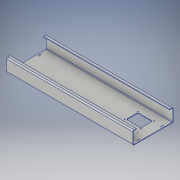
# Autodesk Inventor part: main chassis
Saved by Autodesk Inventor 2018.1 (Build 221171000, 171)
## iProperties
Created: 2018-11-08
Part Number: main chassis
Material: Aluminum 6061
Document SubType Name: Sheet Metal
Designer: RCCol
Density: 2.7 g/cm^3
Sheet Metal Rule: .125 thick aluminum
Appearance: Aluminum - Flat
Author: RCCol
Autodesk Inventor part; units mm, degrees
ref_plane "YZ Plane" through (0, 0, 0) normal (1, 0, 0) x (0, 1, 0)
ref_plane "XZ Plane" through (0, 0, 0) normal (0, 1, 0) x (-1, 0, 0)
ref_plane "XY Plane" through (0, 0, 0) normal (0, 0, 1) x (1, 0, 0)
sketch "Sketch1" plane through (0, 0, 0) normal (0, 1, 0) x (-1, 0, 0)
  line L0 (0, 0) -> (-673.1, 0)
  line L1 (-673.1, 0) -> (-673.1, -215.9)
  line L2 (-673.1, -215.9) -> (0, -215.9)
  line L3 (0, -215.9) -> (0, 0)
  dimension "d0" = 673.1
  dimension "d1" = 215.9
  measures "d0" distance of L2.end L1.end
  measures "d1" distance of L1.end L0.end
extrude "Plate1" add sketch "Sketch1" along normal blind 3.175
sketch "Sketch2" plane through (0, 0, -212.725) normal (0, 0, -1) x (-1, 0, 0)
  line L0 (-673.1, 0) -> (0, 0)
  line L1 (0, 0) -> (0, 69.85)
  line L2 (0, 69.85) -> (-673.1, 69.85)
  line L3 (-673.1, 69.85) -> (-673.1, 0)
  constraints: 6 end point, 1 horizontal, 1 perpendicular, 1 vertical
edge flange "Flange1" height 69.85 angle 90 thickness 3.175 bend radius 3.175 thickness toward (0, 0, -1) relief straight relief width 3.175 relief depth 1.5875 edges at (336.55, 3.175, -215.9) wall of the first edge with corners at (673.1, 0, -212.725) (0, 0, -212.725) (0, 69.85, -212.725) (673.1, 69.85, -212.725)
bend "Bend1"
corner "Corner1"
sketch "Sketch3" plane through (673.1, 0, -3.175) normal (0, 0, 1) x (1, 0, 0)
  line L0 (-673.1, 0) -> (0, 0)
  line L1 (0, 0) -> (0, 69.85)
  line L2 (0, 69.85) -> (-673.1, 69.85)
  line L3 (-673.1, 69.85) -> (-673.1, 0)
  constraints: 6 end point, 1 horizontal, 1 perpendicular, 1 vertical
edge flange "Flange2" height 69.85 angle 90 thickness 3.175 bend radius 3.175 thickness toward (0, 0, 1) relief straight relief width 3.175 relief depth 1.5875 edges at (336.55, 3.175, 0) wall of the first edge with corners at (0, 0, -3.175) (673.1, 0, -3.175) (673.1, 69.85, -3.175) (0, 69.85, -3.175)
bend "Bend2"
corner "Corner2"
sketch "Sketch4" plane through (0, 66.675, -215.9) normal (0, 1, 0) x (-1, 0, 0)
  line L0 (-673.1, 0) -> (0, 0)
  line L1 (0, 0) -> (0, 19.05)
  line L2 (0, 19.05) -> (-673.1, 19.05)
  line L3 (-673.1, 19.05) -> (-673.1, 0)
  constraints: 6 end point, 1 horizontal, 1 perpendicular, 1 vertical
edge flange "Flange3" height 19.05 angle 90 thickness 3.175 bend radius 3.175 thickness toward (0, 1, 0) relief straight relief width 3.175 relief depth 1.5875 corner gap 3.175 corner form 0 edges at (336.55, 69.85, -212.725) (336.55, 69.85, -3.175) wall of the first edge with corners at (673.1, 66.675, -215.9) (0, 66.675, -215.9) (0, 66.675, -196.85) (673.1, 66.675, -196.85)
bend "Bend3"
corner "Corner3"
sketch "A$C12E85A68" plane through (0, 0, 0) normal (0, 0, 1) x (1, 0, 0)
  line L0 (6.985, 0) -> (-6.985, 0)
  point P0 (0, 0)
sketch "A$C3FBB3793" plane through (0, 0, 0) normal (0, 0, 1) x (1, 0, 0)
  line L0 (6.985, 0) -> (-6.985, 0)
  point P0 (0, 0)
sketch "switch" plane through (0, 0, 0) normal (0, 0, 1) x (1, 0, 0)
  circle A0 centre (258.1551, -160.6447) radius 1.9558
  circle A1 centre (258.1551, -132.0697) radius 1.9558
  line L0 (261.3301, -152.7072) -> (254.9801, -152.7072)
  line L1 (254.9801, -152.7072) -> (254.9801, -140.0072)
  line L2 (254.9801, -140.0072) -> (261.3301, -140.0072)
  line L3 (261.3301, -140.0072) -> (261.3301, -152.7072)
  point P0 (0, 0)
sketch "A$C150B116C" plane through (0, 0, 0) normal (0, 0, 1) x (1, 0, 0)
  circle A0 centre (0, -14.2875) radius 1.9558
  circle A1 centre (0, 14.2875) radius 1.9558
  line L0 (3.175, -6.35) -> (-3.175, -6.35)
  line L1 (-3.175, -6.35) -> (-3.175, 6.35)
  line L2 (-3.175, 6.35) -> (3.175, 6.35)
  line L3 (3.175, 6.35) -> (3.175, -6.35)
  point P0 (0, 0)
sketch "A$C47CC5A6E" plane through (0, 0, 0) normal (0, 0, 1) x (1, 0, 0)
  circle A0 centre (0, -14.2875) radius 1.9558
  circle A1 centre (0, 14.2875) radius 1.9558
  line L0 (3.175, -6.35) -> (-3.175, -6.35)
  line L1 (-3.175, -6.35) -> (-3.175, 6.35)
  line L2 (-3.175, 6.35) -> (3.175, 6.35)
  line L3 (3.175, 6.35) -> (3.175, -6.35)
  point P0 (0, 0)
sketch "A$C2A516532" plane through (0, 0, 0) normal (0, 0, 1) x (1, 0, 0)
  circle A0 centre (0, -14.2875) radius 1.9558
  circle A1 centre (0, 14.2875) radius 1.9558
  line L0 (3.175, -6.35) -> (-3.175, -6.35)
  line L1 (-3.175, -6.35) -> (-3.175, 6.35)
  line L2 (-3.175, 6.35) -> (3.175, 6.35)
  line L3 (3.175, 6.35) -> (3.175, -6.35)
  point P0 (0, 0)
sketch "A$C2A9E7CC2" plane through (0, 0, 0) normal (0, 0, 1) x (1, 0, 0)
  circle A0 centre (0, -12.7) radius 4.7625
  circle A1 centre (0, 12.7) radius 4.7625
  circle A2 centre (0, 12.7) radius 4.7625
  circle A3 centre (0, -12.7) radius 4.7625
  point P0 (0, 0)
sketch "A$C56AF9537" plane through (0, 0, 0) normal (0, 0, 1) x (1, 0, 0)
  circle A0 centre (0, 0) radius 4.7625
  circle A1 centre (38.1, 0) radius 4.7625
  circle A2 centre (38.1, 0) radius 4.7625
  circle A3 centre (0, 0) radius 4.7625
sketch "A$C5AAF1D81" plane through (0, 0, 0) normal (0, 0, 1) x (1, 0, 0)
  circle A0 centre (0, 0) radius 4.7625
sketch "A$C295C71F8" plane through (0, 0, 0) normal (0, 0, 1) x (1, 0, 0)
  line L0 (-24.6482, -5.1614) -> (-26.1518, -5.1614)
  arc A0 (-24.6482, -6.1774) -> (-26.1518, -6.1774) centre (-25.4, 0) ccw
  line L1 (-26.1518, -5.1614) -> (-26.1518, -6.1774)
  line L2 (-24.6482, -6.1774) -> (-24.6482, -5.1614)
  line L3 (0.7518, -5.1614) -> (-0.7518, -5.1614)
  arc A1 (0.7518, -6.1774) -> (-0.7518, -6.1774) centre (0, 0) ccw
  line L4 (-0.7518, -5.1614) -> (-0.7518, -6.1774)
  line L5 (0.7518, -6.1774) -> (0.7518, -5.1614)
sketch "A$C1F257043" plane through (0, 0, 0) normal (0, 0, 1) x (1, 0, 0)
  line L0 (-24.6482, -5.1614) -> (-26.1518, -5.1614)
  arc A0 (-24.6482, -6.1774) -> (-26.1518, -6.1774) centre (-25.4, 0) ccw
  line L1 (-26.1518, -5.1614) -> (-26.1518, -6.1774)
  line L2 (-24.6482, -6.1774) -> (-24.6482, -5.1614)
  line L3 (0.7518, -5.1614) -> (-0.7518, -5.1614)
  arc A1 (0.7518, -6.1774) -> (-0.7518, -6.1774) centre (0, 0) ccw
  line L4 (-0.7518, -5.1614) -> (-0.7518, -6.1774)
  line L5 (0.7518, -6.1774) -> (0.7518, -5.1614)
sketch "A$C62022436" plane through (0, 0, 0) normal (0, 0, 1) x (1, 0, 0)
  circle A0 centre (0, 0) radius 3.2004
sketch "A$C5D572602" plane through (0, 0, 0) normal (0, 0, 1) x (1, 0, 0)
  circle A0 centre (237.6, 34.925) radius 15.1
  arc A1 (239.251, 56.7808) -> (238.6557, 57.3761) centre (238.6557, 56.7808) ccw
  arc A2 (238.6557, 52.4739) -> (239.251, 53.0692) centre (238.6557, 53.0692) ccw
  line L0 (239.251, 53.0692) -> (239.251, 56.7808)
  arc A3 (236.5443, 57.3761) -> (235.949, 56.7808) centre (236.5443, 56.7808) ccw
  line L1 (235.949, 53.0692) -> (235.949, 56.7808)
  line L2 (238.6557, 57.3761) -> (236.5443, 57.3761)
  line L3 (238.6557, 52.4739) -> (236.5443, 52.4739)
  arc A4 (235.949, 53.0692) -> (236.5443, 52.4739) centre (236.5443, 53.0692) ccw
  arc A5 (239.251, 16.7808) -> (238.6557, 17.3761) centre (238.6557, 16.7808) ccw
  arc A6 (238.6557, 12.4739) -> (239.251, 13.0692) centre (238.6557, 13.0692) ccw
  line L4 (239.251, 13.0692) -> (239.251, 16.7808)
  arc A7 (236.5443, 17.3761) -> (235.949, 16.7808) centre (236.5443, 16.7808) ccw
  line L5 (235.949, 13.0692) -> (235.949, 16.7808)
  line L6 (238.6557, 17.3761) -> (236.5443, 17.3761)
  line L7 (238.6557, 12.4739) -> (236.5443, 12.4739)
  arc A8 (235.949, 13.0692) -> (236.5443, 12.4739) centre (236.5443, 13.0692) ccw
  circle A9 centre (174.1, 34.925) radius 15.1
  arc A10 (175.751, 56.7808) -> (175.1557, 57.3761) centre (175.1557, 56.7808) ccw
  arc A11 (175.1557, 52.4739) -> (175.751, 53.0692) centre (175.1557, 53.0692) ccw
  line L8 (175.751, 53.0692) -> (175.751, 56.7808)
  arc A12 (173.0443, 57.3761) -> (172.449, 56.7808) centre (173.0443, 56.7808) ccw
  line L9 (172.449, 53.0692) -> (172.449, 56.7808)
  line L10 (175.1557, 57.3761) -> (173.0443, 57.3761)
  line L11 (175.1557, 52.4739) -> (173.0443, 52.4739)
  arc A13 (172.449, 53.0692) -> (173.0443, 52.4739) centre (173.0443, 53.0692) ccw
  arc A14 (175.751, 16.7808) -> (175.1557, 17.3761) centre (175.1557, 16.7808) ccw
  arc A15 (175.1557, 12.4739) -> (175.751, 13.0692) centre (175.1557, 13.0692) ccw
  line L12 (175.751, 13.0692) -> (175.751, 16.7808)
  arc A16 (173.0443, 17.3761) -> (172.449, 16.7808) centre (173.0443, 16.7808) ccw
  line L13 (172.449, 13.0692) -> (172.449, 16.7808)
  line L14 (175.1557, 17.3761) -> (173.0443, 17.3761)
  line L15 (175.1557, 12.4739) -> (173.0443, 12.4739)
  arc A17 (172.449, 13.0692) -> (173.0443, 12.4739) centre (173.0443, 13.0692) ccw
  circle A18 centre (110.6, 34.925) radius 15.1
  arc A19 (112.251, 56.7808) -> (111.6557, 57.3761) centre (111.6557, 56.7808) ccw
  arc A20 (111.6557, 52.4739) -> (112.251, 53.0692) centre (111.6557, 53.0692) ccw
  line L16 (112.251, 53.0692) -> (112.251, 56.7808)
  arc A21 (109.5443, 57.3761) -> (108.949, 56.7808) centre (109.5443, 56.7808) ccw
  line L17 (108.949, 53.0692) -> (108.949, 56.7808)
  line L18 (111.6557, 57.3761) -> (109.5443, 57.3761)
  line L19 (111.6557, 52.4739) -> (109.5443, 52.4739)
  arc A22 (108.949, 53.0692) -> (109.5443, 52.4739) centre (109.5443, 53.0692) ccw
  arc A23 (112.251, 16.7808) -> (111.6557, 17.3761) centre (111.6557, 16.7808) ccw
  arc A24 (111.6557, 12.4739) -> (112.251, 13.0692) centre (111.6557, 13.0692) ccw
  line L20 (112.251, 13.0692) -> (112.251, 16.7808)
  arc A25 (109.5443, 17.3761) -> (108.949, 16.7808) centre (109.5443, 16.7808) ccw
  line L21 (108.949, 13.0692) -> (108.949, 16.7808)
  line L22 (111.6557, 17.3761) -> (109.5443, 17.3761)
  line L23 (111.6557, 12.4739) -> (109.5443, 12.4739)
  arc A26 (108.949, 13.0692) -> (109.5443, 12.4739) centre (109.5443, 13.0692) ccw
  circle A27 centre (47.1, 34.925) radius 15.1
  arc A28 (48.751, 56.7808) -> (48.1557, 57.3761) centre (48.1557, 56.7808) ccw
  arc A29 (48.1557, 52.4739) -> (48.751, 53.0692) centre (48.1557, 53.0692) ccw
  line L24 (48.751, 53.0692) -> (48.751, 56.7808)
  arc A30 (46.0443, 57.3761) -> (45.449, 56.7808) centre (46.0443, 56.7808) ccw
  line L25 (45.449, 53.0692) -> (45.449, 56.7808)
  line L26 (48.1557, 57.3761) -> (46.0443, 57.3761)
  line L27 (48.1557, 52.4739) -> (46.0443, 52.4739)
  arc A31 (45.449, 53.0692) -> (46.0443, 52.4739) centre (46.0443, 53.0692) ccw
  arc A32 (48.751, 16.7808) -> (48.1557, 17.3761) centre (48.1557, 16.7808) ccw
  arc A33 (48.1557, 12.4739) -> (48.751, 13.0692) centre (48.1557, 13.0692) ccw
  line L28 (48.751, 13.0692) -> (48.751, 16.7808)
  arc A34 (46.0443, 17.3761) -> (45.449, 16.7808) centre (46.0443, 16.7808) ccw
  line L29 (45.449, 13.0692) -> (45.449, 16.7808)
  line L30 (48.1557, 17.3761) -> (46.0443, 17.3761)
  line L31 (48.1557, 12.4739) -> (46.0443, 12.4739)
  arc A35 (45.449, 13.0692) -> (46.0443, 12.4739) centre (46.0443, 13.0692) ccw
  circle A36 centre (269.35, 26.3058) radius 1.651
  circle A37 centre (450.85, 36.5125) radius 9.525
  circle A38 centre (440.7472, 46.6153) radius 1.651
  circle A39 centre (460.9528, 26.4097) radius 1.651
  circle A40 centre (412.75, 36.5125) radius 9.525
  circle A41 centre (402.6472, 46.6153) radius 1.651
  circle A42 centre (422.8528, 26.4097) radius 1.651
  circle A43 centre (374.65, 36.5125) radius 9.525
  circle A44 centre (364.5472, 46.6153) radius 1.651
  circle A45 centre (384.7528, 26.4097) radius 1.651
  circle A46 centre (336.55, 36.5125) radius 9.525
  circle A47 centre (326.4472, 46.6153) radius 1.651
  circle A48 centre (346.6528, 26.4097) radius 1.651
  circle A49 centre (298.45, 36.5125) radius 9.525
  circle A50 centre (288.3472, 46.6153) radius 1.651
  circle A51 centre (308.5528, 26.4097) radius 1.651
  circle A52 centre (205.85, 26.3058) radius 1.651
  circle A53 centre (78.85, 26.3058) radius 1.651
  circle A54 centre (142.35, 25.4) radius 1.651
  circle A55 centre (22.225, 19.9558) radius 1.651
  circle A56 centre (217.85, 59.9558) radius 1.65
  circle A57 centre (205.85, 59.9558) radius 4.826
  circle A58 centre (257.35, 58.3683) radius 1.65
  circle A59 centre (281.35, 58.3683) radius 1.65
  circle A60 centre (269.35, 58.3683) radius 4.826
  circle A61 centre (336.55, 20.6375) radius 1.651
  circle A62 centre (450.85, 52.3875) radius 1.651
  circle A63 centre (374.65, 52.3875) radius 1.651
  circle A64 centre (336.55, 52.3875) radius 1.651
  point P0 (0, 0)
sketch "A$C7192318C" plane through (0, 0, 0) normal (0, 0, 1) x (1, 0, 0)
  circle A0 centre (0, 0) radius 9.525
  circle A1 centre (-10.1028, 10.1028) radius 1.651
  circle A2 centre (10.1028, -10.1028) radius 1.651
  circle A3 centre (-38.1, 0) radius 9.525
  circle A4 centre (-48.2028, 10.1028) radius 1.651
  circle A5 centre (-27.9972, -10.1028) radius 1.651
  circle A6 centre (-38.1, -15.875) radius 1.651
  circle A7 centre (0, 15.875) radius 1.651
  circle A8 centre (-38.1, 15.875) radius 1.651
  circle A9 centre (0, -15.875) radius 1.651
  circle A10 centre (0, 15.875) radius 1.651
sketch "A$C1B597E17" plane through (0, 0, 0) normal (0, 0, 1) x (1, 0, 0)
  circle A0 centre (38.1, 0) radius 9.525
  circle A1 centre (27.9972, 10.1028) radius 1.651
  circle A2 centre (48.2028, -10.1028) radius 1.651
  circle A3 centre (0, 0) radius 9.525
  circle A4 centre (-10.1028, 10.1028) radius 1.651
  circle A5 centre (10.1028, -10.1028) radius 1.651
  circle A6 centre (0, -15.875) radius 1.651
  circle A7 centre (38.1, 15.875) radius 1.651
  circle A8 centre (0, 15.875) radius 1.651
  circle A9 centre (38.1, -15.875) radius 1.651
  circle A10 centre (38.1, 15.875) radius 1.651
sketch "IEC" plane through (0, 0, 0) normal (0, 0, 1) x (1, 0, 0)
  circle A0 centre (286.9353, -202.8198) radius 1.651
  line L0 (280.9396, -192.8979) -> (253.2435, -192.8979)
  line L1 (280.9396, -212.7417) -> (253.2435, -212.7417)
  line L2 (253.2435, -192.8979) -> (253.2435, -212.7417)
  circle A1 centre (247.2478, -202.8198) radius 1.651
  line L3 (280.9396, -192.8979) -> (280.9396, -212.7417)
  point P0 (0, 0)
sketch "fuse" plane through (0, 0, 0) normal (0, 0, 1) x (1, 0, 0)
  line L0 (342.1968, -199.5105) -> (342.1968, -206.1291)
  line L1 (353.6268, -199.5105) -> (353.6268, -206.1291)
  arc A0 (353.6268, -199.5105) -> (342.1968, -199.5105) centre (347.9118, -202.8198) ccw
  arc A1 (342.1968, -206.1291) -> (353.6268, -206.1291) centre (347.9118, -202.8198) ccw
  point P0 (0, 0)
sketch "slide switches" plane through (0, 0, 0) normal (0, 0, 1) x (1, 0, 0)
  circle A0 centre (535.1886, -188.5323) radius 1.9558
  circle A1 centre (535.1886, -217.1073) radius 1.9558
  line L0 (532.0136, -196.4698) -> (538.3636, -196.4698)
  line L1 (538.3636, -196.4698) -> (538.3636, -209.1698)
  line L2 (538.3636, -209.1698) -> (532.0136, -209.1698)
  line L3 (532.0136, -209.1698) -> (532.0136, -196.4698)
  circle A2 centre (551.1906, -188.5323) radius 1.9558
  circle A3 centre (551.1906, -217.1073) radius 1.9558
  line L4 (548.0156, -196.4698) -> (554.3656, -196.4698)
  line L5 (554.3656, -196.4698) -> (554.3656, -209.1698)
  line L6 (554.3656, -209.1698) -> (548.0156, -209.1698)
  line L7 (548.0156, -209.1698) -> (548.0156, -196.4698)
  point P0 (0, 0)
sketch "slide switches2" plane through (0, 0, 0) normal (0, 0, 1) x (1, 0, 0)
  circle A0 centre (652.6918, -188.5323) radius 1.9558
  circle A1 centre (652.6918, -217.1073) radius 1.9558
  line L0 (649.5168, -196.4698) -> (655.8668, -196.4698)
  line L1 (655.8668, -196.4698) -> (655.8668, -209.1698)
  line L2 (655.8668, -209.1698) -> (649.5168, -209.1698)
  line L3 (649.5168, -209.1698) -> (649.5168, -196.4698)
  circle A2 centre (668.6938, -188.5323) radius 1.9558
  circle A3 centre (668.6938, -217.1073) radius 1.9558
  line L4 (665.5188, -196.4698) -> (671.8688, -196.4698)
  line L5 (671.8688, -196.4698) -> (671.8688, -209.1698)
  line L6 (671.8688, -209.1698) -> (665.5188, -209.1698)
  line L7 (665.5188, -209.1698) -> (665.5188, -196.4698)
  point P0 (0, 0)
sketch "power switches" plane through (0, 0, 0) normal (0, 0, 1) x (1, 0, 0)
  line L0 (277.5254, 61.1673) -> (279.0291, 61.1673)
  arc A0 (277.5254, 62.1833) -> (279.0291, 62.1833) centre (278.2772, 56.0059) ccw
  line L1 (279.0291, 61.1673) -> (279.0291, 62.1833)
  line L2 (277.5254, 62.1833) -> (277.5254, 61.1673)
  line L3 (252.1254, 61.1673) -> (253.6291, 61.1673)
  arc A1 (252.1254, 62.1833) -> (253.6291, 62.1833) centre (252.8772, 56.0059) ccw
  line L4 (253.6291, 61.1673) -> (253.6291, 62.1833)
  line L5 (252.1254, 62.1833) -> (252.1254, 61.1673)
  point P0 (0, 0)
sketch "A$C18423190" plane through (0, 0, 0) normal (0, 0, 1) x (1, 0, 0)
  circle A0 centre (-32.45, 0) radius 1.651
  circle A1 centre (-13.4, 0) radius 1.651
  circle A2 centre (0, 0) radius 1.651
  circle A3 centre (-45.85, 0) radius 1.651
sketch "circuit board" plane through (0, 0, 0) normal (0, 0, 1) x (1, 0, 0)
  line L0 (389.1697, -271.4536) -> (846.3697, -271.4536)
  line L1 (846.3697, -271.4536) -> (846.3697, -350.8286)
  line L2 (846.3697, -350.8286) -> (389.1697, -350.8286)
  line L3 (389.1697, -350.8286) -> (389.1697, -271.4536)
  line L4 (500.2947, -350.8286) -> (500.3911, -338.129)
  line L5 (566.9697, -350.8286) -> (566.9697, -338.1286)
  line L6 (609.8195, -350.8286) -> (609.8195, -338.1286)
  line L7 (389.1697, -350.8286) -> (635.2195, -350.8286)
  line L8 (635.2195, -350.8286) -> (635.2195, -338.1286)
  line L9 (389.1697, -350.8286) -> (687.6196, -350.9711)
  line L10 (687.6196, -350.9711) -> (687.6196, -338.2711)
  point P0 (0, 0)
  point P1 (487.5653, -332.1944)
  point P2 (557.874, -329.5492)
  point P3 (601.453, -330.6482)
  point P4 (627.1199, -330.3649)
  point P5 (677.3002, -331.9135)
sketch "A$C7C926527" plane through (0, 0, 0) normal (0, 0, 1) x (1, 0, 0)
  line L0 (-0.3193, 63.4992) -> (673.054, 63.4992)
  line L1 (673.0221, -0.0009) -> (0, 0)
  circle A0 centre (536.3135, 31.7496) radius 4.7625
  circle A1 centre (422.0135, 31.7496) radius 4.7625
  circle A2 centre (422.0135, 31.7496) radius 4.7625
  circle A3 centre (536.3135, 31.7496) radius 4.7625
  circle A4 centre (498.2135, 31.7496) radius 4.7625
  circle A5 centre (385.5953, 19.0496) radius 4.7625
  circle A6 centre (385.5953, 44.4496) radius 4.7625
  circle A7 centre (385.5953, 44.4496) radius 4.7625
  circle A8 centre (385.5953, 19.0496) radius 4.7625
  circle A9 centre (266.3903, 31.7496) radius 4.7625
  circle A10 centre (266.3903, 31.7496) radius 4.7625
  circle A11 centre (240.9903, 31.7496) radius 4.7625
  circle A12 centre (240.9903, 31.7496) radius 4.7625
  circle A13 centre (215.5903, 31.7496) radius 4.7625
  circle A14 centre (215.5903, 31.7496) radius 4.7625
  circle A15 centre (100.6236, 31.7496) radius 4.7625
  circle A16 centre (100.6236, 31.7496) radius 4.7625
  circle A17 centre (460.1135, 31.7496) radius 4.7625
  circle A18 centre (460.1135, 31.7496) radius 4.7625
  circle A19 centre (290.9172, 31.7867) radius 3.2004
  line L2 (673.054, 63.4992) -> (673.054, -0.0008)
  line L3 (-0.3193, 63.4992) -> (0, 0)
  circle A20 centre (81.5736, 31.7496) radius 1.016
  circle A21 centre (119.6736, 31.7496) radius 1.016
  circle A22 centre (87.1532, 18.2792) radius 1.016
  circle A23 centre (100.6236, 12.6996) radius 1.016
  circle A24 centre (114.094, 18.2792) radius 1.016
  circle A25 centre (188.6269, 47.6246) radius 3.2385
  circle A26 centre (188.6269, 31.7496) radius 3.2385
  circle A27 centre (188.6269, 15.8746) radius 3.2385
  line L4 (19.004, 63.4992) -> (654.004, 63.4992)
  line L5 (654.004, 63.4992) -> (654.004, 279.3992)
  line L6 (654.004, 279.3992) -> (19.004, 279.3992)
  line L7 (19.004, 279.3992) -> (19.004, 63.4992)
  circle A28 centre (485.7443, 295.1472) radius 3.175
  circle A29 centre (485.7443, 327.1512) radius 3.175
  circle A30 centre (485.7443, 311.1492) radius 3.175
  circle A31 centre (485.7443, 311.1492) radius 3.175
  circle A32 centre (485.7443, 327.1512) radius 3.175
  circle A33 centre (485.7443, 295.1472) radius 3.175
  circle A34 centre (631.7943, 323.8492) radius 4.7625
  circle A35 centre (600.0443, 311.1492) radius 4.7625
  circle A36 centre (561.9443, 311.1492) radius 4.7625
  circle A37 centre (631.7943, 298.4492) radius 4.7625
  circle A38 centre (631.7943, 298.4492) radius 4.7625
  circle A39 centre (561.9443, 311.1492) radius 4.7625
  circle A40 centre (600.0443, 311.1492) radius 4.7625
  circle A41 centre (631.7943, 323.8492) radius 4.7625
  circle A42 centre (523.8443, 311.1492) radius 4.7625
  circle A43 centre (523.8443, 311.1492) radius 4.7625
  circle A44 centre (415.8943, 311.1492) radius 4.7625
  circle A45 centre (301.5943, 311.1492) radius 4.7625
  circle A46 centre (166.426, 31.7496) radius 4.7625
  circle A47 centre (225.3943, 311.1492) radius 4.7625
  circle A48 centre (263.4943, 311.1492) radius 4.7625
  circle A49 centre (339.6943, 311.1492) radius 4.7625
  circle A50 centre (377.7943, 311.1492) radius 4.7625
  circle A51 centre (453.9943, 311.1492) radius 4.7625
  circle A52 centre (453.9943, 311.1492) radius 4.7625
  circle A53 centre (377.7943, 311.1492) radius 4.7625
  circle A54 centre (339.6943, 311.1492) radius 4.7625
  circle A55 centre (263.4943, 311.1492) radius 4.7625
  circle A56 centre (225.3943, 311.1492) radius 4.7625
  circle A57 centre (166.426, 31.7496) radius 4.7625
  circle A58 centre (301.5943, 311.1492) radius 4.7625
  circle A59 centre (415.8943, 311.1492) radius 4.7625
  circle A60 centre (88.8693, 311.1492) radius 3.9624
  circle A61 centre (88.8693, 311.1492) radius 3.9624
  line L8 (673.0693, 279.3992) -> (-0.0307, 279.3992)
  line L9 (-0.0307, 279.3992) -> (-0.0307, 342.8992)
  line L10 (-0.0307, 342.8992) -> (673.0693, 342.8992)
  line L11 (673.0693, 342.8992) -> (673.0693, 279.3992)
  circle A62 centre (78.1917, 104.7055) radius 15.1
  arc A63 (79.8427, 126.5613) -> (79.2474, 127.1566) centre (79.2474, 126.5613) ccw
  arc A64 (79.2474, 122.2544) -> (79.8427, 122.8497) centre (79.2474, 122.8497) ccw
  line L12 (79.8427, 122.8497) -> (79.8427, 126.5613)
  arc A65 (77.136, 127.1566) -> (76.5407, 126.5613) centre (77.136, 126.5613) ccw
  line L13 (76.5407, 122.8497) -> (76.5407, 126.5613)
  line L14 (79.2474, 127.1566) -> (77.136, 127.1566)
  line L15 (79.2474, 122.2544) -> (77.136, 122.2544)
  arc A66 (76.5407, 122.8497) -> (77.136, 122.2544) centre (77.136, 122.8497) ccw
  arc A67 (79.8427, 86.5613) -> (79.2474, 87.1566) centre (79.2474, 86.5613) ccw
  arc A68 (79.2474, 82.2544) -> (79.8427, 82.8497) centre (79.2474, 82.8497) ccw
  line L16 (79.8427, 82.8497) -> (79.8427, 86.5613)
  arc A69 (77.136, 87.1566) -> (76.5407, 86.5613) centre (77.136, 86.5613) ccw
  line L17 (76.5407, 82.8497) -> (76.5407, 86.5613)
  line L18 (79.2474, 87.1566) -> (77.136, 87.1566)
  line L19 (79.2474, 82.2544) -> (77.136, 82.2544)
  arc A70 (76.5407, 82.8497) -> (77.136, 82.2544) centre (77.136, 82.8497) ccw
  circle A71 centre (44.4267, 132.2334) radius 1.651
  circle A72 centre (47.6017, 89.7363) radius 1.651
  circle A73 centre (135.3417, 104.7055) radius 15.1
  arc A74 (136.9927, 126.5613) -> (136.3974, 127.1566) centre (136.3974, 126.5613) ccw
  arc A75 (136.3974, 122.2544) -> (136.9927, 122.8497) centre (136.3974, 122.8497) ccw
  line L20 (136.9927, 122.8497) -> (136.9927, 126.5613)
  arc A76 (134.286, 127.1566) -> (133.6907, 126.5613) centre (134.286, 126.5613) ccw
  line L21 (133.6907, 122.8497) -> (133.6907, 126.5613)
  line L22 (136.3974, 127.1566) -> (134.286, 127.1566)
  line L23 (136.3974, 122.2544) -> (134.286, 122.2544)
  arc A77 (133.6907, 122.8497) -> (134.286, 122.2544) centre (134.286, 122.8497) ccw
  arc A78 (136.9927, 86.5613) -> (136.3974, 87.1566) centre (136.3974, 86.5613) ccw
  arc A79 (136.3974, 82.2544) -> (136.9927, 82.8497) centre (136.3974, 82.8497) ccw
  line L24 (136.9927, 82.8497) -> (136.9927, 86.5613)
  arc A80 (134.286, 87.1566) -> (133.6907, 86.5613) centre (134.286, 86.5613) ccw
  line L25 (133.6907, 82.8497) -> (133.6907, 86.5613)
  line L26 (136.3974, 87.1566) -> (134.286, 87.1566)
  line L27 (136.3974, 82.2544) -> (134.286, 82.2544)
  arc A81 (133.6907, 82.8497) -> (134.286, 82.2544) centre (134.286, 82.8497) ccw
  circle A82 centre (107.2917, 132.2334) radius 1.651
  circle A83 centre (110.4667, 89.7363) radius 1.651
  circle A84 centre (153.5294, 132.3021) radius 1.651
  circle A85 centre (156.7044, 89.805) radius 1.651
  circle A86 centre (216.7633, 94.4988) radius 1.651
  circle A87 centre (229.9883, 104.7055) radius 9.525
  circle A88 centre (219.8855, 114.8083) radius 1.651
  circle A89 centre (240.0911, 94.6027) radius 1.651
  circle A90 centre (229.9883, 88.8305) radius 1.651
  circle A91 centre (229.9883, 120.5805) radius 1.651
  circle A92 centre (254.8633, 94.4988) radius 1.651
  circle A93 centre (268.0883, 104.7055) radius 9.525
  circle A94 centre (257.9855, 114.8083) radius 1.651
  circle A95 centre (278.1911, 94.6027) radius 1.651
  circle A96 centre (268.0883, 88.8305) radius 1.651
  circle A97 centre (268.0883, 120.5805) radius 1.651
  circle A98 centre (292.9633, 94.4988) radius 1.651
  circle A99 centre (306.1883, 104.7055) radius 9.525
  circle A100 centre (296.0855, 114.8083) radius 1.651
  circle A101 centre (316.2911, 94.6027) radius 1.651
  circle A102 centre (306.1883, 88.8305) radius 1.651
  circle A103 centre (306.1883, 120.5805) radius 1.651
  circle A104 centre (350.6383, 104.7055) radius 17.4625
  circle A105 centre (350.6383, 129.3181) radius 1.651
  circle A106 centre (350.6383, 80.0929) radius 1.651
  circle A107 centre (381.8633, 94.4988) radius 1.651
  circle A108 centre (395.0883, 104.7055) radius 9.525
  circle A109 centre (384.9855, 114.8083) radius 1.651
  circle A110 centre (405.1911, 94.6027) radius 1.651
  circle A111 centre (395.0883, 88.8305) radius 1.651
  circle A112 centre (395.0883, 120.5805) radius 1.651
  circle A113 centre (498.2135, 104.7055) radius 15.1
  arc A114 (499.8645, 126.5613) -> (499.2692, 127.1566) centre (499.2692, 126.5613) ccw
  arc A115 (499.2692, 122.2544) -> (499.8645, 122.8497) centre (499.2692, 122.8497) ccw
  line L28 (499.8645, 122.8497) -> (499.8645, 126.5613)
  arc A116 (497.1579, 127.1566) -> (496.5625, 126.5613) centre (497.1579, 126.5613) ccw
  line L29 (496.5625, 122.8497) -> (496.5625, 126.5613)
  line L30 (499.2692, 127.1566) -> (497.1579, 127.1566)
  line L31 (499.2692, 122.2544) -> (497.1579, 122.2544)
  arc A117 (496.5625, 122.8497) -> (497.1579, 122.2544) centre (497.1579, 122.8497) ccw
  arc A118 (499.8645, 86.5613) -> (499.2692, 87.1566) centre (499.2692, 86.5613) ccw
  arc A119 (499.2692, 82.2544) -> (499.8645, 82.8497) centre (499.2692, 82.8497) ccw
  line L32 (499.8645, 82.8497) -> (499.8645, 86.5613)
  arc A120 (497.1579, 87.1566) -> (496.5625, 86.5613) centre (497.1579, 86.5613) ccw
  line L33 (496.5625, 82.8497) -> (496.5625, 86.5613)
  line L34 (499.2692, 87.1566) -> (497.1579, 87.1566)
  line L35 (499.2692, 82.2544) -> (497.1579, 82.2544)
  arc A121 (496.5625, 82.8497) -> (497.1579, 82.2544) centre (497.1579, 82.8497) ccw
  circle A122 centre (548.4885, 94.4988) radius 1.651
  circle A123 centre (561.7135, 104.7055) radius 9.525
  circle A124 centre (551.6108, 114.8083) radius 1.651
  circle A125 centre (571.8163, 94.6027) radius 1.651
  circle A126 centre (561.7135, 88.8305) radius 1.651
  circle A127 centre (561.7135, 120.5805) radius 1.651
  circle A128 centre (592.9385, 94.4988) radius 1.651
  circle A129 centre (606.1635, 104.7055) radius 9.525
  circle A130 centre (596.0608, 114.8083) radius 1.651
  circle A131 centre (616.2663, 94.6027) radius 1.651
  circle A132 centre (606.1635, 88.8305) radius 1.651
  circle A133 centre (606.1635, 120.5805) radius 1.651
  line L36 (-0.0307, 279.3992) -> (-0.3193, 63.4992)
  line L37 (673.0693, 279.3992) -> (673.054, 63.4992)
  circle A134 centre (9.3423, 236.5748) radius 1.5875
  circle A135 centre (9.3423, 229.2342) radius 2.667
  circle A136 centre (9.3423, 221.8936) radius 1.5875
  circle A137 centre (9.3423, 109.5748) radius 1.5875
  circle A138 centre (9.3423, 102.2342) radius 2.667
  circle A139 centre (9.3423, 94.8936) radius 1.5875
  circle A140 centre (663.529, 236.5748) radius 1.5875
  circle A141 centre (663.529, 229.2342) radius 2.667
  circle A142 centre (663.529, 221.8936) radius 1.5875
  circle A143 centre (663.529, 109.5748) radius 1.5875
  circle A144 centre (663.529, 102.2342) radius 2.667
  circle A145 centre (663.529, 94.8936) radius 1.5875
  circle A146 centre (187.2943, 311.1492) radius 4.7625
  line L38 (64.978, 226.4674) -> (128.732, 226.4674)
  arc A147 (136.606, 218.5934) -> (128.732, 226.4674) centre (128.732, 218.5934) ccw
  line L39 (136.606, 218.5934) -> (136.606, 171.8574)
  arc A148 (128.732, 163.9834) -> (136.606, 171.8574) centre (128.732, 171.8574) ccw
  line L40 (128.732, 163.9834) -> (64.978, 163.9834)
  arc A149 (57.104, 171.8574) -> (64.978, 163.9834) centre (64.978, 171.8574) ccw
  line L41 (57.104, 171.8574) -> (57.104, 218.5934)
  arc A150 (64.978, 226.4674) -> (57.104, 218.5934) centre (64.978, 218.5934) ccw
  circle A151 centre (53.167, 160.3004) radius 2.7813
  circle A152 centre (140.543, 160.3004) radius 2.7813
  circle A153 centre (53.167, 230.1504) radius 2.7813
  circle A154 centre (140.543, 230.1504) radius 2.7813
  circle A155 centre (350.5197, 31.7496) radius 4.7625
  circle A156 centre (350.5197, 31.7496) radius 4.7625
  circle A157 centre (315.444, 19.0496) radius 4.7625
  circle A158 centre (315.444, 44.4496) radius 4.7625
  circle A159 centre (315.444, 44.4496) radius 4.7625
  circle A160 centre (315.444, 19.0496) radius 4.7625
  circle A161 centre (162.7108, 143.5787) radius 1.65
  circle A162 centre (162.7108, 232.4787) radius 1.65
  circle A163 centre (200.4933, 207.0787) radius 2.65
  circle A164 centre (200.4933, 246.7662) radius 2.65
  circle A165 centre (251.2933, 155.496) radius 2.65
  circle A166 centre (259.2308, 155.496) radius 2.65
  circle A167 centre (251.2933, 238.046) radius 2.65
  circle A168 centre (259.2308, 238.046) radius 2.65
  circle A169 centre (274.4708, 143.5787) radius 1.65
  circle A170 centre (294.7358, 150.5637) radius 1.65
  circle A171 centre (274.4708, 232.4787) radius 1.65
  circle A172 centre (294.7358, 207.7137) radius 1.65
  arc A173 (202.9933, 237.7568) -> (197.9933, 237.7568) centre (200.4933, 237.7568) ccw
  arc A174 (197.9933, 232.7568) -> (202.9933, 232.7568) centre (200.4933, 232.7568) ccw
  line L42 (202.9933, 237.7568) -> (202.9933, 232.7568)
  line L43 (197.9933, 237.7568) -> (197.9933, 232.7568)
  arc A175 (202.9933, 158.7787) -> (197.9933, 158.7787) centre (200.4933, 158.7787) ccw
  arc A176 (197.9933, 153.7787) -> (202.9933, 153.7787) centre (200.4933, 153.7787) ccw
  line L44 (202.9933, 158.7787) -> (202.9933, 153.7787)
  line L45 (197.9933, 158.7787) -> (197.9933, 153.7787)
  arc A177 (323.4714, 244.2662) -> (323.4714, 249.2662) centre (323.4714, 246.7662) ccw
  arc A178 (316.4714, 249.2662) -> (316.4714, 244.2662) centre (316.4714, 246.7662) ccw
  line L46 (323.4714, 244.2662) -> (316.4714, 244.2662)
  line L47 (323.4714, 249.2662) -> (316.4714, 249.2662)
  arc A179 (258.3839, 244.2662) -> (258.3839, 249.2662) centre (258.3839, 246.7662) ccw
  arc A180 (251.3839, 249.2662) -> (251.3839, 244.2662) centre (251.3839, 246.7662) ccw
  line L48 (258.3839, 244.2662) -> (251.3839, 244.2662)
  line L49 (258.3839, 249.2662) -> (251.3839, 249.2662)
  arc A181 (313.5308, 235.546) -> (313.5308, 240.546) centre (313.5308, 238.046) ccw
  arc A182 (306.5308, 240.546) -> (306.5308, 235.546) centre (306.5308, 238.046) ccw
  line L50 (313.5308, 235.546) -> (306.5308, 235.546)
  line L51 (313.5308, 240.546) -> (306.5308, 240.546)
  arc A183 (323.4714, 178.7662) -> (323.4714, 183.7662) centre (323.4714, 181.2662) ccw
  arc A184 (316.4714, 183.7662) -> (316.4714, 178.7662) centre (316.4714, 181.2662) ccw
  line L52 (323.4714, 178.7662) -> (316.4714, 178.7662)
  line L53 (323.4714, 183.7662) -> (316.4714, 183.7662)
  arc A185 (323.4714, 168.0662) -> (323.4714, 173.0662) centre (323.4714, 170.5662) ccw
  arc A186 (316.4714, 173.0662) -> (316.4714, 168.0662) centre (316.4714, 170.5662) ccw
  line L54 (323.4714, 168.0662) -> (316.4714, 168.0662)
  line L55 (323.4714, 173.0662) -> (316.4714, 173.0662)
  arc A187 (258.3839, 178.7662) -> (258.3839, 183.7662) centre (258.3839, 181.2662) ccw
  arc A188 (251.3839, 183.7662) -> (251.3839, 178.7662) centre (251.3839, 181.2662) ccw
  line L56 (258.3839, 178.7662) -> (251.3839, 178.7662)
  line L57 (258.3839, 183.7662) -> (251.3839, 183.7662)
  arc A189 (258.3839, 168.0662) -> (258.3839, 173.0662) centre (258.3839, 170.5662) ccw
  arc A190 (251.3839, 173.0662) -> (251.3839, 168.0662) centre (251.3839, 170.5662) ccw
  line L58 (258.3839, 168.0662) -> (251.3839, 168.0662)
  line L59 (258.3839, 173.0662) -> (251.3839, 173.0662)
  arc A191 (313.5308, 152.996) -> (313.5308, 157.996) centre (313.5308, 155.496) ccw
  arc A192 (306.5308, 157.996) -> (306.5308, 152.996) centre (306.5308, 155.496) ccw
  line L60 (313.5308, 152.996) -> (306.5308, 152.996)
  line L61 (313.5308, 157.996) -> (306.5308, 157.996)
  circle A193 centre (175.0933, 174.6715) radius 4.8
  circle A194 centre (227.5358, 161.846) radius 4.8
  circle A195 centre (324.8926, 203.6662) radius 6.35
  circle A196 centre (249.9626, 203.6662) radius 6.35
  arc A197 (202.9933, 172.788) -> (197.9933, 172.788) centre (200.4933, 172.788) ccw
  arc A198 (197.9933, 167.788) -> (202.9933, 167.788) centre (200.4933, 167.788) ccw
  line L62 (202.9933, 172.788) -> (202.9933, 167.788)
  line L63 (197.9933, 172.788) -> (197.9933, 167.788)
  circle A199 centre (625.4628, 162.0207) radius 1.65
  circle A200 centre (625.4628, 219.1707) radius 1.65
  circle A201 centre (592.1253, 242.3482) radius 1.651
  circle A202 centre (547.6753, 251.8732) radius 1.651
  circle A203 centre (611.1753, 242.3482) radius 1.651
  circle A204 centre (566.7253, 251.8732) radius 1.651
  circle A205 centre (580.1253, 251.8732) radius 1.651
  circle A206 centre (534.2753, 251.8732) radius 1.651
  circle A207 centre (527.0378, 158.0507) radius 4.826
  circle A208 centre (501.6378, 158.0507) radius 4.826
  circle A209 centre (556.1906, 172.1807) radius 2.3813
  circle A210 centre (595.7958, 192.3606) radius 2.3813
  circle A211 centre (538.6893, 187.2568) radius 6.35
  circle A212 centre (583.5567, 207.2078) radius 2.3813
  circle A213 centre (476.4253, 251.8732) radius 1.651
  circle A214 centre (495.4753, 251.8732) radius 1.651
  circle A215 centre (508.8753, 251.8732) radius 1.651
  circle A216 centre (463.0253, 251.8732) radius 1.651
  circle A217 centre (72.1121, 31.7496) radius 1.651
  line L64 (66.1164, 21.8277) -> (38.4203, 21.8277)
  line L65 (66.1164, 41.6715) -> (38.4203, 41.6715)
  line L66 (38.4203, 21.8277) -> (38.4203, 41.6715)
  circle A218 centre (32.4246, 31.7496) radius 1.651
  line L67 (66.1164, 21.8277) -> (66.1164, 41.6715)
  line L68 (133.0885, 28.4403) -> (133.0885, 35.0589)
  line L69 (144.5185, 28.4403) -> (144.5185, 35.0589)
  arc A219 (144.5185, 28.4403) -> (133.0885, 28.4403) centre (138.8035, 31.7496) cw
  arc A220 (133.0885, 35.0589) -> (144.5185, 35.0589) centre (138.8035, 31.7496) cw
  line L70 (62.7175, 316.3106) -> (64.2211, 316.3106)
  arc A221 (62.7175, 317.3266) -> (64.2211, 317.3266) centre (63.4693, 311.1492) ccw
  line L71 (64.2211, 316.3106) -> (64.2211, 317.3266)
  line L72 (62.7175, 317.3266) -> (62.7175, 316.3106)
  line L73 (37.3175, 316.3106) -> (38.8211, 316.3106)
  arc A222 (37.3175, 317.3266) -> (38.8211, 317.3266) centre (38.0693, 311.1492) ccw
  line L74 (38.8211, 316.3106) -> (38.8211, 317.3266)
  line L75 (37.3175, 317.3266) -> (37.3175, 316.3106)
  line L76 (174.3464, 228.2284) -> (631.5464, 228.2284)
  line L77 (631.5464, 228.2284) -> (631.5464, 148.8534)
  line L78 (631.5464, 148.8534) -> (174.3464, 148.8534)
  line L79 (174.3464, 148.8534) -> (174.3464, 228.2284)
  line L80 (285.4714, 148.8534) -> (285.5679, 161.553)
  line L81 (352.1464, 148.8534) -> (352.1464, 161.5534)
  line L82 (394.9962, 148.8534) -> (394.9962, 161.5534)
  line L83 (174.3464, 148.8534) -> (420.3962, 148.8534)
  line L84 (420.3962, 148.8534) -> (420.3962, 161.5534)
  line L85 (174.3464, 148.8534) -> (472.7964, 148.711)
  line L86 (472.7964, 148.711) -> (472.7964, 161.411)
  point P0 (272.7421, 167.4876)
  point P1 (343.0508, 170.1328)
  point P2 (386.6298, 169.0338)
  point P3 (412.2967, 169.3171)
  point P4 (462.4769, 167.7685)
sketch "Sketch5" plane through (0, 0, 0) normal (0, -1, 0) x (1, 0, 0)
  line L0 (673.3733, 0) -> (0, 0)
  line L1 (654.05, 0) -> (19.05, 0)
  line L2 (19.05, 0) -> (19.05, -215.9)
  line L3 (19.05, -215.9) -> (654.05, -215.9)
  line L4 (654.05, -215.9) -> (654.05, 0)
  line L5 (-0.0153, -215.9) -> (673.0847, -215.9)
  circle A0 centre (566.3129, -41.2063) radius 15.1
  arc A1 (564.6619, -63.0621) -> (565.2572, -63.6574) centre (565.2572, -63.0621) ccw
  arc A2 (565.2572, -58.7552) -> (564.6619, -59.3505) centre (565.2572, -59.3505) ccw
  line L6 (564.6619, -59.3505) -> (564.6619, -63.0621)
  arc A3 (567.3686, -63.6574) -> (567.9639, -63.0621) centre (567.3686, -63.0621) ccw
  line L7 (567.9639, -59.3505) -> (567.9639, -63.0621)
  line L8 (565.2572, -63.6574) -> (567.3686, -63.6574)
  line L9 (565.2572, -58.7552) -> (567.3686, -58.7552)
  arc A4 (567.9639, -59.3505) -> (567.3686, -58.7552) centre (567.3686, -59.3505) ccw
  arc A5 (564.6619, -23.0621) -> (565.2572, -23.6574) centre (565.2572, -23.0621) ccw
  arc A6 (565.2572, -18.7552) -> (564.6619, -19.3505) centre (565.2572, -19.3505) ccw
  line L10 (564.6619, -19.3505) -> (564.6619, -23.0621)
  arc A7 (567.3686, -23.6574) -> (567.9639, -23.0621) centre (567.3686, -23.0621) ccw
  line L11 (567.9639, -19.3505) -> (567.9639, -23.0621)
  line L12 (565.2572, -23.6574) -> (567.3686, -23.6574)
  line L13 (565.2572, -18.7552) -> (567.3686, -18.7552)
  arc A8 (567.9639, -19.3505) -> (567.3686, -18.7552) centre (567.3686, -19.3505) ccw
  circle A9 centre (628.6273, -68.7342) radius 1.651
  circle A10 centre (625.4523, -26.2371) radius 1.651
  circle A11 centre (502.188, -41.2063) radius 15.1
  arc A12 (500.537, -63.0621) -> (501.1323, -63.6574) centre (501.1323, -63.0621) ccw
  arc A13 (501.1323, -58.7552) -> (500.537, -59.3505) centre (501.1323, -59.3505) ccw
  line L14 (500.537, -59.3505) -> (500.537, -63.0621)
  arc A14 (503.2437, -63.6574) -> (503.839, -63.0621) centre (503.2437, -63.0621) ccw
  line L15 (503.839, -59.3505) -> (503.839, -63.0621)
  line L16 (501.1323, -63.6574) -> (503.2437, -63.6574)
  line L17 (501.1323, -58.7552) -> (503.2437, -58.7552)
  arc A15 (503.839, -59.3505) -> (503.2437, -58.7552) centre (503.2437, -59.3505) ccw
  arc A16 (500.537, -23.0621) -> (501.1323, -23.6574) centre (501.1323, -23.0621) ccw
  arc A17 (501.1323, -18.7552) -> (500.537, -19.3505) centre (501.1323, -19.3505) ccw
  line L18 (500.537, -19.3505) -> (500.537, -23.0621)
  arc A18 (503.2437, -23.6574) -> (503.839, -23.0621) centre (503.2437, -23.0621) ccw
  line L19 (503.839, -19.3505) -> (503.839, -23.0621)
  line L20 (501.1323, -23.6574) -> (503.2437, -23.6574)
  line L21 (501.1323, -18.7552) -> (503.2437, -18.7552)
  arc A19 (503.839, -19.3505) -> (503.2437, -18.7552) centre (503.2437, -19.3505) ccw
  circle A20 centre (534.0379, -26.2371) radius 1.651
  circle A21 centre (443.0657, -41.2063) radius 9.525
  circle A22 centre (443.0657, -25.3313) radius 1.651
  circle A23 centre (443.0657, -57.0813) radius 1.651
  circle A24 centre (404.9657, -41.2063) radius 9.525
  circle A25 centre (404.9657, -25.3313) radius 1.651
  circle A26 centre (404.9657, -57.0813) radius 1.651
  circle A27 centre (366.8657, -41.2063) radius 9.525
  circle A28 centre (366.8657, -25.3313) radius 1.651
  circle A29 centre (366.8657, -57.0813) radius 1.651
  circle A30 centre (319.2407, -41.2063) radius 17.4625
  circle A31 centre (319.2407, -65.8189) radius 1.651
  circle A32 centre (319.2407, -16.5937) radius 1.651
  circle A33 centre (271.6157, -41.2063) radius 9.525
  circle A34 centre (271.6157, -25.3313) radius 1.651
  circle A35 centre (271.6157, -57.0813) radius 1.651
  circle A36 centre (174.8405, -41.2063) radius 15.1
  arc A37 (173.1895, -63.0621) -> (173.7848, -63.6574) centre (173.7848, -63.0621) ccw
  arc A38 (173.7848, -58.7552) -> (173.1895, -59.3505) centre (173.7848, -59.3505) ccw
  line L22 (173.1895, -59.3505) -> (173.1895, -63.0621)
  arc A39 (175.8962, -63.6574) -> (176.4915, -63.0621) centre (175.8962, -63.0621) ccw
  line L23 (176.4915, -59.3505) -> (176.4915, -63.0621)
  line L24 (173.7848, -63.6574) -> (175.8962, -63.6574)
  line L25 (173.7848, -58.7552) -> (175.8962, -58.7552)
  arc A40 (176.4915, -59.3505) -> (175.8962, -58.7552) centre (175.8962, -59.3505) ccw
  arc A41 (173.1895, -23.0621) -> (173.7848, -23.6574) centre (173.7848, -23.0621) ccw
  arc A42 (173.7848, -18.7552) -> (173.1895, -19.3505) centre (173.7848, -19.3505) ccw
  line L26 (173.1895, -19.3505) -> (173.1895, -23.0621)
  arc A43 (175.8962, -23.6574) -> (176.4915, -23.0621) centre (175.8962, -23.0621) ccw
  line L27 (176.4915, -19.3505) -> (176.4915, -23.0621)
  line L28 (173.7848, -23.6574) -> (175.8962, -23.6574)
  line L29 (173.7848, -18.7552) -> (175.8962, -18.7552)
  arc A44 (176.4915, -19.3505) -> (175.8962, -18.7552) centre (175.8962, -19.3505) ccw
  circle A45 centre (111.3405, -41.2063) radius 9.525
  circle A46 centre (111.3405, -25.3313) radius 1.651
  circle A47 centre (111.3405, -57.0813) radius 1.651
  circle A48 centre (66.8905, -41.2063) radius 9.525
  circle A49 centre (66.8905, -25.3313) radius 1.651
  circle A50 centre (66.8905, -57.0813) radius 1.651
  line L30 (673.0847, -215.9) -> (673.3733, 0)
  line L31 (-0.0153, -215.9) -> (0, 0)
  line L32 (608.076, -162.9682) -> (544.322, -162.9682)
  arc A51 (536.448, -155.0942) -> (544.322, -162.9682) centre (544.322, -155.0942) ccw
  line L33 (536.448, -155.0942) -> (536.448, -108.3582)
  arc A52 (544.322, -100.4842) -> (536.448, -108.3582) centre (544.322, -108.3582) ccw
  line L34 (544.322, -100.4842) -> (608.076, -100.4842)
  arc A53 (615.95, -108.3582) -> (608.076, -100.4842) centre (608.076, -108.3582) ccw
  line L35 (615.95, -108.3582) -> (615.95, -155.0942)
  arc A54 (608.076, -162.9682) -> (615.95, -155.0942) centre (608.076, -155.0942) ccw
  circle A55 centre (619.887, -96.8012) radius 2.7813
  circle A56 centre (532.511, -96.8012) radius 2.7813
  circle A57 centre (619.887, -166.6512) radius 2.7813
  circle A58 centre (532.511, -166.6512) radius 2.7813
  circle A59 centre (9.525, -46.0756) radius 1.5875
  circle A60 centre (9.525, -38.735) radius 2.667
  circle A61 centre (9.525, -31.3944) radius 1.5875
  circle A62 centre (663.7117, -173.0756) radius 1.5875
  circle A63 centre (663.7117, -165.735) radius 2.667
  circle A64 centre (663.7117, -158.3944) radius 1.5875
  circle A65 centre (663.7117, -46.0756) radius 1.5875
  circle A66 centre (663.7117, -38.735) radius 2.667
  circle A67 centre (663.7117, -31.3944) radius 1.5875
  circle A68 centre (9.525, -173.0756) radius 1.5875
  circle A69 centre (9.525, -165.735) radius 2.667
  circle A70 centre (9.525, -158.3944) radius 1.5875
  circle A71 centre (608.076, -155.0942) radius 7.874
  circle A72 centre (544.322, -155.0942) radius 7.874
  circle A73 centre (544.322, -108.3582) radius 7.874
  circle A74 centre (608.076, -108.3582) radius 7.874
  line L36 (608.076, -162.9682) -> (544.322, -162.9682)
  line L37 (544.322, -162.9682) -> (544.322, -100.4842)
  line L38 (544.322, -100.4842) -> (608.076, -100.4842)
  line L39 (608.076, -100.4842) -> (608.076, -162.9682)
  line L40 (536.448, -108.3582) -> (615.95, -108.3582)
  line L41 (615.95, -108.3582) -> (615.95, -155.0942)
  line L42 (615.95, -155.0942) -> (536.448, -155.0942)
  line L43 (536.448, -155.0942) -> (536.448, -108.3582)
  circle A75 centre (503.2437, -63.0621) radius 0.5953
  circle A76 centre (501.1323, -63.0621) radius 0.5953
  circle A77 centre (501.1323, -59.3505) radius 0.5953
  circle A78 centre (503.2437, -59.3505) radius 0.5953
  line L44 (503.839, -63.6574) -> (500.537, -63.6574)
  line L45 (500.537, -63.6574) -> (500.537, -58.7552)
  line L46 (500.537, -58.7552) -> (503.839, -58.7552)
  line L47 (503.839, -58.7552) -> (503.839, -63.6574)
  line L48 (503.839, -23.6803) -> (500.537, -23.6803)
  line L49 (500.537, -23.6803) -> (500.537, -18.7552)
  line L50 (500.537, -18.7552) -> (503.839, -18.7552)
  line L51 (503.839, -18.7552) -> (503.839, -23.6803)
  line L52 (564.6619, -18.7552) -> (567.9639, -18.7552)
  line L53 (567.9639, -18.7552) -> (567.9639, -23.6803)
  line L54 (567.9639, -23.6803) -> (564.6619, -23.6803)
  line L55 (564.6619, -23.6803) -> (564.6619, -18.7552)
  line L56 (567.9639, -63.6574) -> (564.6619, -63.6574)
  line L57 (564.6619, -63.6574) -> (564.6619, -58.7552)
  line L58 (564.6619, -58.7552) -> (567.9639, -58.7552)
  line L59 (567.9639, -58.7552) -> (567.9639, -63.6574)
  line L60 (173.1895, -58.7552) -> (176.4915, -58.7552)
  line L61 (176.4915, -58.7552) -> (176.4915, -63.6574)
  line L62 (176.4915, -63.6574) -> (173.1895, -63.6574)
  line L63 (173.1895, -63.6574) -> (173.1895, -58.7552)
  line L64 (173.1895, -18.7552) -> (176.4915, -18.7552)
  line L65 (176.4915, -18.7552) -> (176.4915, -23.6803)
  line L66 (176.4915, -23.6803) -> (173.1895, -23.6803)
  line L67 (173.1895, -23.6803) -> (173.1895, -18.7552)
  point P0 (9.525, -31.3944)
  point P1 (663.7117, -165.735)
  point P2 (663.7117, -158.3944)
  point P3 (663.7117, -46.0756)
  point P4 (663.7117, -38.735)
  point P5 (663.7117, -31.3944)
  point P6 (9.525, -173.0756)
  point P7 (9.525, -165.735)
  point P8 (9.525, -158.3944)
  point P9 (9.525, -46.0756)
  point P10 (663.7117, -173.0756)
  point P11 (9.525, -38.735)
  constraints: 136 end point, 78 centre point, 56 point on circle, 16 parallel, 15 point on line, 8 coincident, 8 horizontal, 8 perpendicular, 3 concentric, 1 vertical alignment, 3 other
extrude "Cut1" cut sketch "Sketch5" against normal blind 3.175 contours A0 | L6 A2 L9 A4 L7 A3 L8 A1 | A1 L56 L57 | L57 L58 A2 | A3 L59 L56 | L58 L59 A4 | L10 A6 L13 A8 L11 A7 L12 A5 | A5 L12 A7 L53 L54 L55 | L55 L52 A6 | L52 L53 A8 | A9 | A10 | A11 | A76 A12 | L14 A77 L17 A78 L15 A75 L16 A76 | A12 L44 L45 | L45 L46 A13 | A13 A77 | A75 A14 | A14 L47 L44 | L46 L47 A15 | A15 A78 | L18 A17 L21 A19 L19 A18 L20 A16 | A16 L20 A18 L51 L48 L49 | L49 L50 A17 | L50 L51 A19 | A20 | A21 | A22 | A23 | A24 | A25 | A26 | A27 | A28 | A29 | A30 | A31 | A32 | A33 | A34 | A35 | A36 | L22 A38 L25 A40 L23 A39 L24 A37 | A37 L62 L63 | L63 L60 A38 | A39 L61 L62 | L60 L61 A40 | L26 A42 L29 A44 L27 A43 L28 A41 | A41 L28 A43 L65 L66 L67 | L67 L64 A42 | L64 L65 A44 | A45 | A46 | A47 | A48 | A49 | A50 | L39 L42 A54 | L32 A72 L42 A71 | A71 L42 L39 | L37 L42 A72 | A51 L42 L37 | A71 L39 A74 L35 | L42 L39 A71 | L42 A72 L37 A73 L40 A74 L39 A71 | A71 L39 L42 | L33 A73 L37 A72 | A72 L37 L42 | L42 L37 A72 | L40 L39 A53 | A74 L39 L40 | L40 L37 A73 | A52 L37 L40 | A74 L40 A73 L34 | L39 L40 A74 | A74 L40 L39 | A73 L40 L37 | L37 L40 A73 | A55 | A56 | A57 | A58 | A59 | A60 | A61 | A62 | A63 | A64 | A65 | A66 | A67 | A68 | A69 | A70
equation "\"d33\" = Thickness"
equation "\"d2\" = Thickness"
equation "\"d3\" = BendReliefWidth"
equation "\"d4\" = BendReliefDepth"
equation "\"d5\" = MinimumRemnant"
equation "\"d6\" = TransitionRadius"
equation "\"d9\" = BendRadius"
equation "\"d10\" = CornerReliefSize"
equation "\"d11\" = GapSize"
equation "\"d12\" = JacobiRadiusSize"
equation "\"d13\" = BendReliefWidth"
equation "\"d14\" = BendReliefDepth"
equation "\"d15\" = MinimumRemnant"
equation "\"d16\" = TransitionRadius"
equation "\"d19\" = BendRadius"
equation "\"d20\" = CornerReliefSize"
equation "\"d21\" = GapSize"
equation "\"d22\" = JacobiRadiusSize"
equation "\"d23\" = BendReliefWidth"
equation "\"d24\" = BendReliefDepth"
equation "\"d25\" = MinimumRemnant"
equation "\"d26\" = TransitionRadius"
equation "\"d29\" = BendRadius"
equation "\"d30\" = CornerReliefSize"
equation "\"d31\" = GapSize"
equation "\"d32\" = JacobiRadiusSize"
equation "\"BendRadius\" = Thickness"
equation "\"BendReliefWidth\" = Thickness"
equation "\"BendReliefDepth\" = 0.5 * Thickness"
equation "\"CornerReliefSize\" = 4 * Thickness"
equation "\"MinimumRemnant\" = 2 * Thickness"
equation "\"TransitionRadius\" = BendRadius"
equation "\"JacobiRadiusSize\" = BendRadius"
equation "\"GapSize\" = Thickness"
equation "\"Thickness\" = 3.175"
body "Solid1"
